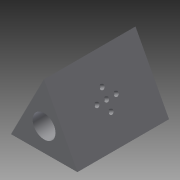
# Autodesk Inventor part: Triangle
Saved by Autodesk Inventor 2014 (Build 180170000, 170)
## iProperties
Created: 2014-03-20
Part Number: Triangle
Material: Generic
Document SubType Name: Modeling
Designer: Pranav
Density: 1 g/cm^3
Appearance: Default
Author: Pranav
Autodesk Inventor part; units mm, degrees
ref_plane "YZ Plane" through (0, 0, 0) normal (1, 0, 0) x (0, 1, 0)
ref_plane "XZ Plane" through (0, 0, 0) normal (0, 1, 0) x (-1, 0, 0)
ref_plane "XY Plane" through (0, 0, 0) normal (0, 0, 1) x (1, 0, 0)
sketch "Sketch1" plane through (0, 0, 0) normal (0, 0, 1) x (1, 0, 0)
  circle A0 centre (0, 0) radius 4.7625
  line L0 (0, 0) -> (-0.0721, 14.2871)
  circle A1 centre (0, 0) radius 16.8508
  line L1 (-13.7645, -9.7205) -> (13.862, -9.581)
  line L2 (-13.7645, -9.7205) -> (-0.0851, 16.8506)
  line L3 (13.862, -9.581) -> (-0.0851, 16.8506)
  dimension "d0" = 9.525
  constraints: 8 end point, 3 point on circle, 2 centre point, 2 coincident, 1 perpendicular, 1 point on line
  measures "d0" diameter of A0
extrude "Extrusion1" add sketch "Sketch1" along normal blind 38.1 contours L3 L1 L2
sketch "Sketch2" plane through (-0.0851, 16.8506, 38.1) normal (0.8844259, 0.4666806, 0) x (0, 0, -1)
  circle A0 centre (19.05, -14.9428) radius 1
  circle A1 centre (19.05, -10.9428) radius 1
  circle A2 centre (19.05, -18.9428) radius 1
  circle A3 centre (23.05, -14.9428) radius 1
  circle A4 centre (15.05, -14.9428) radius 1
  point P0 (38.1, -14.9428)
  dimension "d6" = 2
  dimension "d8" = 2
  dimension "d10" = 2
  dimension "d12" = 2
  dimension "d14" = 2
  constraints: 5 centre point
  measures "d6" diameter of A0
  measures "d8" diameter of A1
  measures "d10" diameter of A2
  measures "d12" diameter of A3
  measures "d14" diameter of A4
extrude "Extrusion2" cut sketch "Sketch2" against normal blind 2
body "Solid1"
